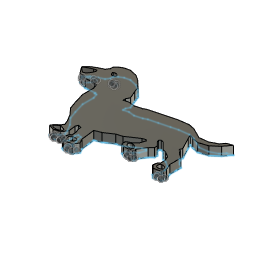
Dog (Autodesk Fusion 360 design; units mm, degrees)
Autodesk Fusion 360 part; units mm, degrees
sketch "Dog" plane through (0, 0, 0) normal (0, 0, 1) x (1, 0, 0)
  line L0 (91, 72) -> (91.5, 72.5)
  line L1 (91.5, 72.5) -> (92.1, 72.85)
  line L2 (92.1, 72.85) -> (92.65, 73.1)
  line L3 (92.65, 73.1) -> (92.9, 73.5)
  line L4 (92.9, 73.5) -> (92.9, 73.8)
  line L5 (92.9, 73.8) -> (93.2, 74.1)
  line L6 (93.2, 74.1) -> (93.6453, 74.3598)
  line L7 (93.6453, 74.3598) -> (94.244, 74.5019)
  line L8 (94.244, 74.5019) -> (95.1334, 74.292)
  line L9 (95.1334, 74.292) -> (95.7, 73.9)
  line L10 (95.7, 73.9) -> (96.0774, 73.5428)
  line L11 (96.0774, 73.5428) -> (96.2166, 73.4111)
  line L12 (96.2166, 73.4111) -> (96.1931, 73.3114)
  line L13 (96.1931, 73.3114) -> (96.4654, 73.1756)
  line L14 (96.4654, 73.1756) -> (96.6, 72.8)
  line L15 (96.6, 72.8) -> (96.6856, 72.5611)
  line L16 (96.6856, 72.5611) -> (96.8, 72.3)
  line L17 (96.8, 72.3) -> (96.936, 71.9896)
  line L18 (96.936, 71.9896) -> (97.0674, 71.6895)
  line L19 (97.0674, 71.6895) -> (96.868, 71.2897)
  line L20 (96.868, 71.2897) -> (96.868, 71)
  line L21 (96.868, 71) -> (97.4262, 71.1448)
  line L22 (97.4262, 71.1448) -> (98.099, 71.0724)
  line L23 (98.099, 71.0724) -> (98.9, 71.3)
  line L24 (98.9, 71.3) -> (99.3, 71.5)
  line L25 (99.3, 71.5) -> (100.2773, 71.7536)
  line L26 (100.2773, 71.7536) -> (101.4237, 72.0511)
  line L27 (101.4237, 72.0511) -> (102.1892, 72.2497)
  line L28 (102.1892, 72.2497) -> (103.3, 72.4)
  line L29 (103.3, 72.4) -> (103.9785, 72.2497)
  line L30 (103.9785, 72.2497) -> (104.6761, 71.9023)
  line L31 (104.6761, 71.9023) -> (105.1731, 71.6549)
  line L32 (105.1731, 71.6549) -> (106.1701, 71.7786)
  line L33 (106.1701, 71.7786) -> (107, 72.2)
  line L34 (107, 72.2) -> (107.4, 72.7)
  line L35 (107.4, 72.7) -> (108, 72.9)
  line L36 (108, 72.9) -> (107.4, 72.1)
  line L37 (107.4, 72.1) -> (106.6, 71.4)
  line L38 (106.6, 71.4) -> (105.6038, 71.0679)
  line L39 (105.6038, 71.0679) -> (104.8565, 71.234)
  line L40 (104.8565, 71.234) -> (104.4, 71.4)
  line L41 (104.4, 71.4) -> (104.6282, 70.9296)
  line L42 (104.6282, 70.9296) -> (105.2301, 69.7891)
  line L43 (105.2301, 69.7891) -> (105.3406, 69.5798)
  line L44 (105.3406, 69.5798) -> (105.2301, 69.2761)
  line L45 (105.2301, 69.2761) -> (105.4321, 69.2026)
  line L46 (105.4321, 69.2026) -> (105.5389, 69.0003)
  line L47 (105.5389, 69.0003) -> (105.7562, 68.7921)
  line L48 (105.7562, 68.7921) -> (106.2, 68.5)
  line L49 (106.2, 68.5) -> (106.2, 68)
  line L50 (106.2, 68) -> (106.2, 67.2)
  line L51 (106.2, 67.2) -> (106.5, 66.5)
  line L52 (106.5, 66.5) -> (106.5, 66.1642)
  line L53 (106.5, 66.1642) -> (106.4122, 65.9833)
  line L54 (106.4122, 65.9833) -> (105.9195, 65.8812)
  line L55 (105.9195, 65.8812) -> (105.5911, 65.8132)
  line L56 (105.5911, 65.8132) -> (105.4637, 65.9322)
  line L57 (105.4637, 65.9322) -> (105.4057, 66.0349)
  line L58 (105.4057, 66.0349) -> (105.2313, 66.1108)
  line L59 (105.2313, 66.1108) -> (105.3185, 66.6056)
  line L60 (105.3185, 66.6056) -> (105.5, 66.8)
  line L61 (105.5, 66.8) -> (105.5, 67.3)
  line L62 (105.5, 67.3) -> (105.2749, 67.8387)
  line L63 (105.2749, 67.8387) -> (104.7, 68.2)
  line L64 (104.7, 68.2) -> (104.3, 68.3)
  line L65 (104.3, 68.3) -> (103.8822, 68.7139)
  line L66 (103.8822, 68.7139) -> (103.5059, 69.0867)
  line L67 (103.5059, 69.0867) -> (103.2191, 69.1584)
  line L68 (103.2191, 69.1584) -> (103.0626, 69.0004)
  line L69 (103.0626, 69.0004) -> (103.1408, 68.7793)
  line L70 (103.1408, 68.7793) -> (103.4021, 68.5204)
  line L71 (103.4021, 68.5204) -> (103.5761, 68.348)
  line L72 (103.5761, 68.348) -> (103.5761, 68)
  line L73 (103.5761, 68) -> (103.2019, 67.6222)
  line L74 (103.2019, 67.6222) -> (102.8, 67)
  line L75 (102.8, 67) -> (102.6382, 66.7495)
  line L76 (102.6382, 66.7495) -> (102.7191, 66.5603)
  line L77 (102.7191, 66.5603) -> (102.5801, 66.4116)
  line L78 (102.5801, 66.4116) -> (102.1432, 66.3211)
  line L79 (102.1432, 66.3211) -> (101.6, 66.3211)
  line L80 (101.6, 66.3211) -> (101.2477, 66.4859)
  line L81 (101.2477, 66.4859) -> (101.2477, 66.9)
  line L82 (101.2477, 66.9) -> (101.8, 67.2)
  line L83 (101.8, 67.2) -> (102.2, 67.6)
  line L84 (102.2, 67.6) -> (102.4, 68.2)
  line L85 (102.4, 68.2) -> (102.2644, 68.3356)
  line L86 (102.2644, 68.3356) -> (101.9, 68.2)
  line L87 (101.9, 68.2) -> (101.4537, 67.9)
  line L88 (101.4537, 67.9) -> (100.5589, 67.2984)
  line L89 (100.5589, 67.2984) -> (99.9, 67.1)
  line L90 (99.9, 67.1) -> (98.9319, 66.4492)
  line L91 (98.9319, 66.4492) -> (98.2267, 66.1869)
  line L92 (98.2267, 66.1869) -> (98.3, 65.6)
  line L93 (98.3, 65.6) -> (98.4261, 64.5909)
  line L94 (98.4261, 64.5909) -> (98.7, 64.1)
  line L95 (98.7, 64.1) -> (98.5631, 63.8652)
  line L96 (98.5631, 63.8652) -> (98.3631, 63.5224)
  line L97 (98.3631, 63.5224) -> (97.8458, 63.4577)
  line L98 (97.8458, 63.4577) -> (97.416, 63.404)
  line L99 (97.416, 63.404) -> (97.2, 63.5)
  line L100 (97.2, 63.5) -> (97.1407, 63.9745)
  line L101 (97.1407, 63.9745) -> (97.2, 64.3)
  line L102 (97.2, 64.3) -> (97.416, 64.4688)
  line L103 (97.416, 64.4688) -> (97.3514, 64.9859)
  line L104 (97.3514, 64.9859) -> (97.2, 65.4)
  line L105 (97.2, 65.4) -> (97.1578, 65.7378)
  line L106 (97.1578, 65.7378) -> (96.8, 65.8)
  line L107 (96.8, 65.8) -> (96.7, 65.5)
  line L108 (96.7, 65.5) -> (96.7597, 65.0219)
  line L109 (96.7597, 65.0219) -> (96.8, 64.6998)
  line L110 (96.8, 64.6998) -> (96.4, 64.1)
  line L111 (96.4, 64.1) -> (95.7, 63.9)
  line L112 (95.7, 63.9) -> (95.1, 64.1)
  line L113 (95.1, 64.1) -> (95.2552, 64.3999)
  line L114 (95.2552, 64.3999) -> (95.7, 64.8)
  line L115 (95.7, 64.8) -> (95.9, 65.1)
  line L116 (95.9, 65.1) -> (95.7, 65.6)
  line L117 (95.7, 65.6) -> (95.2467, 66.3501)
  line L118 (95.2467, 66.3501) -> (94.5812, 67.0899)
  line L119 (94.5812, 67.0899) -> (94.2643, 67.9756)
  line L120 (94.2643, 67.9756) -> (93.9, 69.2)
  line L121 (93.9, 69.2) -> (93.9, 70.5)
  line L122 (93.9, 70.5) -> (93.7194, 71.0048)
  line L123 (93.7194, 71.0048) -> (93.5, 71.0048)
  line L124 (93.5, 71.0048) -> (93.5, 71.1)
  line L125 (93.5, 71.1) -> (92.4041, 71.0048)
  line L126 (92.4041, 71.0048) -> (91.5, 71.3)
  line L127 (91.5, 71.3) -> (91, 72)
  spline S0 degree 5 poles (93.4573, 73.245) (93.4639, 73.2508) (93.4789, 73.262) (93.5069, 73.2776) (93.5543, 73.2951) (93.6255, 73.3096) (93.7021, 73.3144) (93.7773, 73.3081) (93.8452, 73.2897) (93.9021, 73.2598) (93.9465, 73.2202) (93.9782, 73.1737) (93.9977, 73.1233) (94.0059, 73.072) (94.0026, 73.0226) (93.9872, 72.9774) (93.9591, 72.9382) (93.9183, 72.9063) (93.866, 72.8829) (93.8054, 72.8689) (93.7412, 72.8648) (93.6785, 72.8708) (93.622, 72.8867) (93.5748, 72.9116) (93.5376, 72.9441) (93.5086, 72.9819) (93.485, 73.0229) (93.4642, 73.0647) (93.4454, 73.1056) (93.4302, 73.1445) (93.4232, 73.181) (93.428, 73.2081) (93.4394, 73.2272) (93.4508, 73.2392) (93.4573, 73.245) knots 0 0 0 0 0 0 0.033333 0.066667 0.1 0.133333 0.166667 0.2 0.233333 0.266667 0.3 0.333333 0.366667 0.4 0.433333 0.466667 0.5 0.533333 0.566667 0.6 0.633333 0.666667 0.7 0.733333 0.766667 0.8 0.833333 0.866667 0.9 0.933333 0.966667 1 1 1 1 1 1
  spline S1 degree 5 poles (95.8, 64.7) (95.7865, 64.6971) (95.7586, 64.689) (95.7147, 64.6695) (95.6521, 64.63) (95.5713, 64.5651) (95.4935, 64.4941) (95.4245, 64.4263) (95.3698, 64.369) (95.3327, 64.3246) (95.3141, 64.2908) (95.3138, 64.2629) (95.3308, 64.2358) (95.364, 64.2062) (95.4125, 64.1739) (95.4757, 64.1411) (95.5526, 64.1109) (95.6418, 64.0876) (95.7411, 64.0749) (95.8475, 64.076) (95.9572, 64.0931) (96.0661, 64.1268) (96.1691, 64.1764) (96.2612, 64.2388) (96.3364, 64.3084) (96.3896, 64.3781) (96.4162, 64.4406) (96.4141, 64.4902) (96.384, 64.5243) (96.3304, 64.5451) (96.2612, 64.5589) (96.1854, 64.5729) (96.1107, 64.5934) (96.0425, 64.6228) (95.9813, 64.6574) (95.9239, 64.6889) (95.8773, 64.7042) (95.8399, 64.7062) (95.8135, 64.7029) (95.8, 64.7) knots 0 0 0 0 0 0 0.028571 0.057143 0.085714 0.114286 0.142857 0.171429 0.2 0.228571 0.257143 0.285714 0.314286 0.342857 0.371429 0.4 0.428571 0.457143 0.485714 0.514286 0.542857 0.571429 0.6 0.628571 0.657143 0.685714 0.714286 0.742857 0.771429 0.8 0.828571 0.857143 0.885714 0.914286 0.942857 0.971429 1 1 1 1 1 1
  spline S2 degree 5 poles (97.6, 64.3) (97.5781, 64.2934) (97.5366, 64.2785) (97.4819, 64.2512) (97.4265, 64.2062) (97.3865, 64.1383) (97.3733, 64.0625) (97.3824, 63.9829) (97.4091, 63.9039) (97.4494, 63.8302) (97.5004, 63.7664) (97.5597, 63.7166) (97.6259, 63.6846) (97.6985, 63.6726) (97.7777, 63.682) (97.8632, 63.7127) (97.9534, 63.7632) (98.0441, 63.8306) (98.1277, 63.9105) (98.1935, 63.997) (98.2303, 64.0838) (98.2291, 64.1645) (98.185, 64.2334) (98.1001, 64.2862) (97.9843, 64.3204) (97.8512, 64.3346) (97.7432, 64.33) (97.668, 64.3181) (97.6219, 64.3066) (97.6, 64.3) knots 0 0 0 0 0 0 0.04 0.08 0.12 0.16 0.2 0.24 0.28 0.32 0.36 0.4 0.44 0.48 0.52 0.56 0.6 0.64 0.68 0.72 0.76 0.8 0.84 0.88 0.92 0.96 1 1 1 1 1 1
  spline S3 degree 5 poles (101.9447, 67.0876) (101.9232, 67.0894) (101.8808, 67.0908) (101.82, 67.086) (101.747, 67.0664) (101.674, 67.0229) (101.6222, 66.9648) (101.5932, 66.8972) (101.5873, 66.8253) (101.6035, 66.7536) (101.6401, 66.6859) (101.6945, 66.6255) (101.7639, 66.5753) (101.845, 66.5374) (101.9347, 66.5133) (102.0295, 66.5042) (102.1252, 66.5106) (102.2169, 66.5324) (102.2988, 66.5691) (102.364, 66.6192) (102.4054, 66.681) (102.4174, 66.7515) (102.3969, 66.827) (102.3444, 66.9027) (102.2647, 66.9728) (102.1651, 67.0313) (102.0768, 67.0645) (102.01, 67.08) (101.9662, 67.0858) (101.9447, 67.0876) knots 0 0 0 0 0 0 0.04 0.08 0.12 0.16 0.2 0.24 0.28 0.32 0.36 0.4 0.44 0.48 0.52 0.56 0.6 0.64 0.68 0.72 0.76 0.8 0.84 0.88 0.92 0.96 1 1 1 1 1 1
  spline S4 degree 5 poles (105.75, 66.7) (105.7327, 66.696) (105.6998, 66.6855) (105.6561, 66.6626) (105.6102, 66.6191) (105.5726, 66.549) (105.5524, 66.4708) (105.5468, 66.392) (105.5539, 66.3187) (105.574, 66.255) (105.6082, 66.2031) (105.658, 66.164) (105.7239, 66.1381) (105.8042, 66.1253) (105.8951, 66.1259) (105.991, 66.1397) (106.0851, 66.1667) (106.1701, 66.2061) (106.2384, 66.2571) (106.2832, 66.3179) (106.2988, 66.3862) (106.282, 66.4589) (106.2325, 66.5318) (106.1546, 66.5997) (106.0564, 66.6564) (105.9483, 66.6961) (105.8628, 66.7102) (105.8036, 66.7095) (105.7673, 66.704) (105.75, 66.7) knots 0 0 0 0 0 0 0.04 0.08 0.12 0.16 0.2 0.24 0.28 0.32 0.36 0.4 0.44 0.48 0.52 0.56 0.6 0.64 0.68 0.72 0.76 0.8 0.84 0.88 0.92 0.96 1 1 1 1 1 1
  spline S5 degree 5 poles (91.9512, 72.4472) (91.9791, 72.4582) (92.0321, 72.4784) (92.1027, 72.5026) (92.1781, 72.5225) (92.2445, 72.5279) (92.2888, 72.5157) (92.3169, 72.4868) (92.3306, 72.4396) (92.328, 72.3702) (92.3057, 72.2752) (92.2605, 72.154) (92.1916, 72.0116) (92.1026, 71.8602) (91.9992, 71.7162) (91.8886, 71.5966) (91.7776, 71.5161) (91.6717, 71.4843) (91.5731, 71.5014) (91.4803, 71.5572) (91.3906, 71.636) (91.3022, 71.7207) (91.216, 71.7969) (91.1387, 71.8576) (91.083, 71.9062) (91.0631, 71.9507) (91.0906, 72.0008) (91.1704, 72.0634) (91.2965, 72.1387) (91.4557, 72.2226) (91.6309, 72.3081) (91.7692, 72.3713) (91.8647, 72.4124) (91.9233, 72.4363) (91.9512, 72.4472) knots 0 0 0 0 0 0 0.033333 0.066667 0.1 0.133333 0.166667 0.2 0.233333 0.266667 0.3 0.333333 0.366667 0.4 0.433333 0.466667 0.5 0.533333 0.566667 0.6 0.633333 0.666667 0.7 0.733333 0.766667 0.8 0.833333 0.866667 0.9 0.933333 0.966667 1 1 1 1 1 1
  point P0 (93.8, 73.3)
  point P1 (94, 73.1)
  point P2 (93.9, 72.9)
  point P3 (93.6, 72.9)
  point P4 (93.4573, 73.0802)
  point P5 (95.4, 64.4)
  point P6 (95.3286, 64.2429)
  point P7 (95.6, 64.1)
  point P8 (96.2, 64.2)
  point P9 (96.4, 64.5)
  point P10 (96.1, 64.6)
  point P11 (97.3837, 63.9988)
  point P12 (97.6, 63.7)
  point P13 (98, 63.8)
  point P14 (98.2, 64.2)
  point P15 (101.6, 66.9)
  point P16 (101.7477, 66.5902)
  point P17 (102.2041, 66.5327)
  point P18 (102.4, 66.8)
  point P19 (105.55, 66.4)
  point P20 (105.7, 66.15)
  point P21 (106.15, 66.2)
  point P22 (106.25, 66.5)
  point P23 (92.3, 72.5)
  point P24 (92.2607, 72.1628)
  point P25 (91.7, 71.5)
  point P26 (91.2388, 71.7756)
  point P27 (91.1, 72)
  constraint vertical L4
  constraint parallel L1 L6
  constraint parallel L10 L11
  constraint perpendicular L8 L12
  constraint parallel L14 L15
  constraint parallel L16 L17
  constraint parallel L17 L18
  constraint perpendicular L13 L19
  constraint vertical L20
  constraint parallel L21 L25
  constraint parallel L25 L26
  constraint parallel L26 L27
  constraint parallel L30 L31
  constraint parallel L35 L38
  constraint perpendicular L40 L44
  constraint perpendicular L44 L45
  constraint parallel L43 L46
  constraint vertical L49
  constraint parallel L49 L50
  constraint parallel L50 L52
  constraint parallel L54 L55
  constraint vertical L61
  constraint parallel L65 L66
  constraint parallel L64 L67
  constraint perpendicular L66 L68
  constraint perpendicular L68 L70
  constraint perpendicular L68 L71
  constraint vertical L72
  constraint parallel L68 L73
  constraint parallel L74 L75
  constraint perpendicular L56 L77
  constraint parallel L55 L78
  constraint horizontal L79
  constraint perpendicular L79 L81
  constraint perpendicular L83 L85
  constraint parallel L87 L88
  constraint parallel L88 L90
  constraint parallel L86 L91
  constraint parallel L92 L93
  constraint parallel L95 L96
  constraint perpendicular L93 L97
  constraint perpendicular L93 L98
  constraint perpendicular L98 L100
  constraint perpendicular L98 L103
  constraint parallel L103 L105
  constraint parallel L105 L108
  constraint parallel L108 L109
  constraint perpendicular L114 L118
  constraint vertical L121
  constraint parallel L119 L122
  constraint horizontal L123
  constraint perpendicular L123 L124
extrude "Extrude3" add sketch "Dog" along normal blind 1
extrude "Extrude1" [suppressed]
extrude "Extrude2" [suppressed]
named bodies: "dog"
